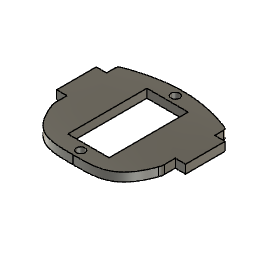
part_A23 (Autodesk Fusion 360 design; units mm, degrees)
Autodesk Fusion 360 part; units mm, degrees
sketch "Sketch1" plane through (0, 0, 0) normal (0, 0, 1) x (1, 0, 0)
  line L0 (0, 0) -> (37.5, 0)
  line L1 (37.5, 0) -> (37.5, 32)
  line L2 (37.5, 32) -> (0, 32)
  line L3 (0, 32) -> (0, 0)
  dimension "d1" = 37.5
  dimension "d2" = 32
  constraint horizontal L0
  constraint vertical L1
  constraint horizontal L2
  constraint vertical L3
  constraint coincident L0.start L3.end
  measures "d1" distance of L0.start L0.end
  measures "d2" distance of L0.start L2.end
extrude "Extrude1" add sketch "Sketch1" along normal blind 2.5
sketch "Sketch2" plane through (0, 0, 2.5) normal (0, 0, 1) x (-1, 0, 0)
  line L0 (0, -32) -> (0, 0)
  line L1 (0, 0) -> (-37.5, 0)
  line L2 (-37.5, 0) -> (-37.5, -32)
  line L3 (-37.5, -32) -> (0, -32)
  circle A0 centre (-18.75, -29.75) radius 1.25
  dimension "d5" = 2.5
  dimension "d6" = 18.75
  dimension "d7" = 2.25
  measures "d5" diameter of A0
  measures "d6" distance of L0 A0.centre
  measures "d7" distance of L3 A0.centre
extrude "Extrude2" cut sketch "Sketch2" against normal blind 3 contours A0
sketch "Sketch3" plane through (0, 0, 2.5) normal (0, 0, 1) x (-1, 0, 0)
  circle A0 centre (-18.75, -29.75) radius 1.25
  line L0 (0, -32) -> (0, 0)
  line L1 (0, 0) -> (-37.5, 0)
  line L2 (-37.5, 0) -> (-37.5, -32)
  line L3 (-37.5, -32) -> (0, -32)
  circle A1 centre (-18.75, -2.25) radius 1.25
  dimension "d10" = 2.5
  dimension "d11" = 27.5
  dimension "d12" = 18.75
  measures "d10" diameter of A1
  measures "d11" vertical distance of A0.centre A1.centre
  measures "d12" distance of L0 A1.centre
extrude "Extrude3" cut sketch "Sketch3" against normal blind 3 contours A1
sketch "Sketch4" plane through (0, 0, 2.5) normal (0, 0, 1) x (-1, 0, 0)
  circle A0 centre (-18.75, -2.25) radius 1.25
  circle A1 centre (-18.75, -29.75) radius 1.25
  line L0 (0, -32) -> (0, 0)
  line L1 (0, 0) -> (-37.5, 0)
  line L2 (-37.5, 0) -> (-37.5, -32)
  line L3 (-37.5, -32) -> (0, -32)
  line L4 (-12.75, -27.5) -> (-24.75, -27.5)
  line L5 (-24.75, -27.5) -> (-24.75, -4.5)
  line L6 (-24.75, -4.5) -> (-12.75, -4.5)
  line L7 (-12.75, -4.5) -> (-12.75, -27.5)
  dimension "d15" = 23
  dimension "d16" = 12
  dimension "d17" = 6
  dimension "d18" = 2.25
  constraint horizontal L4
  constraint vertical L5
  constraint horizontal L6
  constraint vertical L7
  measures "d15" distance of L4.end L5.end
  measures "d16" distance of L4.start L4.end
  measures "d17" distance of A1.centre L7
  measures "d18" distance of A0.centre L6
extrude "Extrude4" cut sketch "Sketch4" against normal blind 3 contours L4 L5 L6 L7
sketch "Sketch5" plane through (37.5, 0, 0) normal (1, 0, 0) x (0, 1, 0)
  line L0 (0, 0) -> (32, 0)
  line L1 (32, 0) -> (32, 2.5)
  line L2 (32, 2.5) -> (0, 2.5)
  line L3 (0, 2.5) -> (0, 0)
  line L4 (25.5, 2.5) -> (14, 2.5)
  line L5 (14, 2.5) -> (14, 0)
  line L6 (14, 0) -> (25.5, 0)
  line L7 (25.5, 0) -> (25.5, 2.5)
  point P0 (27.5, 2.5)
  dimension "d21" = 11.5
  dimension "d22" = 2
  constraint horizontal L4
  constraint vertical L5
  constraint horizontal L6
  constraint vertical L7
  constraint coincident L2 L4.start
  measures "d21" distance of L4.start L4.end
  measures "d22" distance of L7 P0
extrude "Extrude5" cut sketch "Sketch5" against normal blind 3 contours L0 L2 L3 L5 | L0 L1 L2 L7
sketch "Sketch6" plane through (0, 0, 0) normal (-1, 0, 0) x (0, -1, 0)
  line L0 (-32, 0) -> (0, 0)
  line L1 (0, 0) -> (0, 2.5)
  line L2 (0, 2.5) -> (-32, 2.5)
  line L3 (-32, 2.5) -> (-32, 0)
  line L4 (-25.5, 2.5) -> (-14, 2.5)
  line L5 (-14, 2.5) -> (-14, 0)
  line L6 (-14, 0) -> (-25.5, 0)
  line L7 (-25.5, 0) -> (-25.5, 2.5)
  point P0 (-27.5, 2.5)
  dimension "d25" = 11.5
  dimension "d26" = 2
  constraint horizontal L4
  constraint vertical L5
  constraint horizontal L6
  constraint vertical L7
  constraint coincident L2 L4.start
  measures "d25" distance of L4.start L4.end
  measures "d26" distance of L7 P0
extrude "Extrude6" cut sketch "Sketch6" against normal blind 3 contours L0 L2 L3 L7 | L0 L1 L2 L5
sketch "Sketch7" plane through (0, 0, 2.5) normal (0, 0, 1) x (-1, 0, 0)
  line L0 (-3, -25.5) -> (0, -25.5)
  line L1 (0, -25.5) -> (0, -14)
  line L2 (0, -14) -> (-3, -14)
  line L3 (-3, -14) -> (-3, 0)
  line L4 (-3, 0) -> (-34.5, 0)
  line L5 (-34.5, 0) -> (-34.5, -14)
  line L6 (-34.5, -14) -> (-37.5, -14)
  line L7 (-37.5, -14) -> (-37.5, -25.5)
  line L8 (-37.5, -25.5) -> (-34.5, -25.5)
  line L9 (-34.5, -25.5) -> (-34.5, -32)
  line L10 (-34.5, -32) -> (-3, -32)
  line L11 (-3, -32) -> (-3, -25.5)
  circle A0 centre (-18.75, -29.75) radius 1.25
  circle A1 centre (-18.75, -2.25) radius 1.25
  line L12 (-24.75, -27.5) -> (-24.75, -4.5)
  line L13 (-24.75, -4.5) -> (-12.75, -4.5)
  line L14 (-12.75, -4.5) -> (-12.75, -27.5)
  line L15 (-12.75, -27.5) -> (-24.75, -27.5)
  spline S0 degree 5 poles (-3, -28.75) (-3.63, -28.9965) (-4.89, -29.468) (-6.78, -30.1106) (-9.3, -30.8362) (-12.45, -31.5094) (-15.6, -31.9281) (-18.75, -32.0715) (-21.9, -31.9281) (-25.05, -31.5094) (-28.2, -30.8362) (-30.72, -30.1106) (-32.61, -29.468) (-33.87, -28.9965) (-34.5, -28.75) knots 0 0 0 0 0 0 0.1 0.2 0.3 0.4 0.5 0.6 0.7 0.8 0.9 1 1 1 1 1 1
  point P0 (-18.75, -32)
  constraint midpoint L11 S0.start
  constraint midpoint L10 P0
  constraint midpoint L9 S0.end
extrude "Extrude7" cut sketch "Sketch7" against normal blind 3 contours L10 L11 S0 | L9 L10 S0
fillet "Fillet1" radius 1 1 edges at (34.5, 28.75, 1.25)
fillet "Fillet2" radius 1 1 edges at (3, 28.75, 1.25)
sketch "Sketch8" plane through (0, 0, 2.5) normal (0, 0, 1) x (-1, 0, 0)
  spline S0 degree 3 poles (-3, -28.063) (-3, -28.1932) (-3.0254, -28.3222) (-3.1243, -28.5631) (-3.1968, -28.6728) (-3.3388, -28.8166) (-3.3947, -28.8622) (-3.5154, -28.9407) (-3.5797, -28.9732) (-3.647, -28.9986) knots 0 0 0 0 0.039064 0.039064 0.078129 0.078129 0.099711 0.099711 0.121294 0.121294 0.121294 0.121294
  line L0 (-3, -28.063) -> (-3, -25.5)
  line L1 (-3, -25.5) -> (0, -25.5)
  line L2 (0, -25.5) -> (0, -14)
  line L3 (0, -14) -> (-3, -14)
  line L4 (-3, -14) -> (-3, 0)
  line L5 (-3, 0) -> (-34.5, 0)
  line L6 (-34.5, 0) -> (-34.5, -14)
  line L7 (-34.5, -14) -> (-37.5, -14)
  line L8 (-37.5, -14) -> (-37.5, -25.5)
  line L9 (-37.5, -25.5) -> (-34.5, -25.5)
  line L10 (-34.5, -25.5) -> (-34.5, -28.063)
  spline S1 degree 3 poles (-33.853, -28.9986) (-33.9748, -28.9527) (-34.0865, -28.8834) (-34.277, -28.7058) (-34.354, -28.5993) (-34.4385, -28.4156) (-34.4615, -28.3472) (-34.4922, -28.2067) (-34.5, -28.1349) (-34.5, -28.063) knots 0 0 0 0 0.039064 0.039064 0.078129 0.078129 0.099711 0.099711 0.121294 0.121294 0.121294 0.121294
  spline S2 degree 5 poles (-33.853, -28.9986) (-33.3524, -29.1875) (-32.2218, -29.5986) (-30.4612, -30.1847) (-28.0706, -30.8638) (-25.05, -31.5094) (-22.53, -31.8444) (-20.64, -31.9717) (-19.38, -32) (-18.75, -32) knots -0.979459 -0.979459 -0.979459 -0.979459 -0.979459 -0.979459 -0.9 -0.8 -0.7 -0.6 -0.5 -0.5 -0.5 -0.5 -0.5 -0.5
  spline S3 degree 5 poles (-18.75, -32) (-18.12, -32) (-16.86, -31.9717) (-14.97, -31.8444) (-12.45, -31.5094) (-9.4294, -30.8638) (-7.0388, -30.1847) (-5.2782, -29.5986) (-4.1476, -29.1875) (-3.647, -28.9986) knots -0.5 -0.5 -0.5 -0.5 -0.5 -0.5 -0.4 -0.3 -0.2 -0.1 -0.020541 -0.020541 -0.020541 -0.020541 -0.020541 -0.020541
  circle A0 centre (-18.75, -29.75) radius 1.25
  circle A1 centre (-18.75, -2.25) radius 1.25
  line L11 (-24.75, -27.5) -> (-24.75, -4.5)
  line L12 (-24.75, -4.5) -> (-12.75, -4.5)
  line L13 (-12.75, -4.5) -> (-12.75, -27.5)
  line L14 (-12.75, -27.5) -> (-24.75, -27.5)
  spline S4 degree 5 poles (-3, -10.0882) (-3.192, -9.5306) (-3.5896, -8.4564) (-4.2262, -6.9676) (-5.156, -5.2287) (-6.4542, -3.4672) (-7.8881, -2.1125) (-9.4541, -1.1457) (-11.1442, -0.5279) (-12.9429, -0.19) (-14.8281, -0.0435) (-16.7736, -0.0017) (-18.75, 0.0027) (-20.7264, -0.0017) (-22.6719, -0.0435) (-24.5571, -0.19) (-26.3558, -0.5279) (-28.0459, -1.1457) (-29.6119, -2.1125) (-31.0458, -3.4672) (-32.344, -5.2287) (-33.2738, -6.9676) (-33.9104, -8.4564) (-34.308, -9.5306) (-34.5, -10.0882) knots 0 0 0 0 0 0 0.05 0.1 0.15 0.2 0.25 0.3 0.35 0.4 0.45 0.5 0.55 0.6 0.65 0.7 0.75 0.8 0.85 0.9 0.95 1 1 1 1 1 1
  point P0 (-10, -1)
  point P1 (-18.75, 0)
  point P2 (-27.5, -1)
  dimension "d35" = 8.75
  dimension "d36" = 8.75
  dimension "d37" = 1
  dimension "d38" = 1
  constraint coincident L4 S4.start
  constraint midpoint L5 P1
  constraint coincident L6 S4.end
  measures "d35" horizontal distance of P0 P1
  measures "d36" horizontal distance of P1 P2
  measures "d37" distance of L5 P2
  measures "d38" distance of L5 P0
extrude "Extrude8" cut sketch "Sketch8" against normal blind 3 contours L4 L5 S4 | L5 L6 S4
fillet "Fillet3" radius 4 1 edges at (3, 10.0882, 1.25)
fillet "Fillet4" radius 4 1 edges at (34.5, 10.0882, 1.25)
